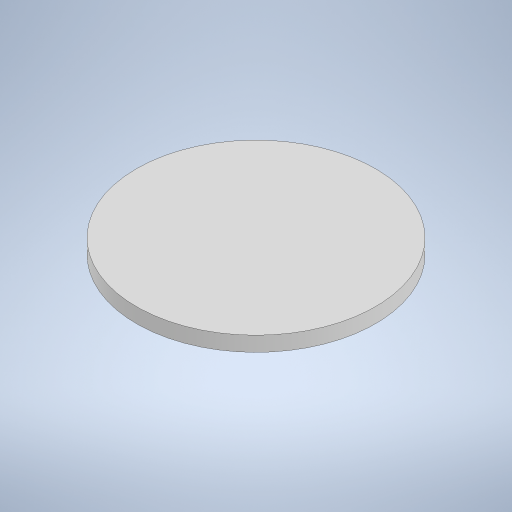
# Autodesk Inventor part: flow director r1
Saved by Autodesk Inventor 2024.1 (Build 281209000, 209)
## iProperties
Created: 2024-08-24
Part Number: flow director r1
Material: Generic
Document SubType Name: Modeling
Designer: pab2
Density: 1 g/cm^3
Appearance: Default
Author: pab2
Autodesk Inventor part; units mm, degrees
ref_plane "YZ Plane" through (0, 0, 0) normal (1, 0, 0) x (0, 1, 0)
ref_plane "XZ Plane" through (0, 0, 0) normal (0, 1, 0) x (-1, 0, 0)
ref_plane "XY Plane" through (0, 0, 0) normal (0, 0, 1) x (1, 0, 0)
sketch "Sketch1" plane through (0, 0, 0) normal (0, 1, 0) x (-1, 0, 0)
  circle A0 centre (0, 0) radius 12.7
  dimension "d0" = 25.4
  constraints: 1 centre point, 1 coincident
  measures "d0" diameter of A0
extrude "Extrusion1" add sketch "Sketch1" along normal blind 1.5748
sketch "Sketch2" plane through (0, 0, 0) normal (0, -1, 0) x (1, 0, 0)
  circle A0 centre (0, 0) radius 9.271
  line L0 (0, -9.271) -> (0, -7.271)
  line L1 (9.271, 0) -> (8.271, 0)
  line L2 (8.271, 0) -> (7.771, 0)
  line L3 (7.771, 0) -> (6.771, 0)
  line L4 (6.771, 0) -> (6.271, 0)
  line L5 (6.271, 0) -> (5.271, 0)
  line L6 (5.271, 0) -> (4.771, 0)
  line L7 (4.771, 0) -> (3.771, 0)
  line L8 (3.771, 0) -> (3.271, 0)
  line L9 (3.271, 0) -> (2.271, 0)
  line L10 (2.271, 0) -> (1.771, 0)
  line L11 (1.771, 0) -> (0.771, 0)
  line L12 (0.771, 0) -> (0.271, 0)
  line L13 (0, 9.271) -> (0, 7.271)
  circle A1 centre (0, 9.271) radius 1
  circle A2 centre (0, -9.271) radius 1
  circle A3 centre (5.7519, 7.271) radius 1
  line L14 (0, 0) -> (-0.5, 0)
  line L15 (-0.5, 0) -> (-1, 0)
  line L16 (-1, 0) -> (-2, 0)
  line L17 (-2, 0) -> (-2.5, 0)
  line L18 (-2.5, 0) -> (-3.5, 0)
  line L19 (-3.5, 0) -> (-4, 0)
  line L20 (-4, 0) -> (-5, 0)
  line L21 (-5, 0) -> (-5.5, 0)
  line L22 (-5.5, 0) -> (-6.5, 0)
  line L23 (-6.5, 0) -> (-7, 0)
  line L24 (-7, 0) -> (-8, 0)
  arc A4 (0, -9.271) -> (5.7519, 7.271) centre (-1.7377, 0.6042) ccw
  arc A5 (0, -9.271) -> (5.7519, 7.271) centre (-2.8108, 0.9773) ccw
  arc A6 (0, -9.271) -> (5.7519, 7.271) centre (-5.6528, 1.9656) ccw
  arc A7 (0, -9.271) -> (5.7519, 7.271) centre (-7.6502, 2.6601) ccw
  arc A8 (0, -9.271) -> (5.7519, 7.271) centre (-14.2057, 4.9395) ccw
  arc A9 (0, -9.271) -> (5.7519, 7.271) centre (-20.4184, 7.0998) ccw
  arc A10 (0, -9.271) -> (5.7519, 7.271) centre (-65.5254, 22.784) ccw
  arc A11 (0, -9.271) -> (5.7519, 7.271) centre (-794.5968, 276.2917) ccw
  arc A12 (5.7519, 7.271) -> (0, -9.271) centre (42.405, -14.7448) ccw
  arc A13 (5.7519, 7.271) -> (0, -9.271) centre (28.5048, -9.9115) ccw
  arc A14 (5.7519, 7.271) -> (0, -9.271) centre (17.401, -6.0506) ccw
  arc A15 (5.7519, 7.271) -> (0, -9.271) centre (14.5425, -5.0566) ccw
  arc A16 (5.7519, 7.271) -> (0, -9.271) centre (11.5077, -4.0014) ccw
  arc A17 (5.7519, 7.271) -> (0, -9.271) centre (10.0566, -3.4968) ccw
  arc A18 (5.7519, 7.271) -> (0, -9.271) centre (7.8443, -2.7276) ccw
  arc A19 (5.7519, 7.271) -> (0, -9.271) centre (6.9625, -2.4209) ccw
  arc A20 (5.7519, 7.271) -> (0, -9.271) centre (5.4808, -1.9057) ccw
  arc A21 (5.7519, 7.271) -> (0, -9.271) centre (4.8418, -1.6836) ccw
  arc A22 (5.7519, 7.271) -> (0, -9.271) centre (3.7059, -1.2886) ccw
  arc A23 (5.7519, 7.271) -> (0, -9.271) centre (3.1926, -1.1101) ccw
  arc A24 (5.7519, 7.271) -> (0, -9.271) centre (2.2472, -0.7814) ccw
  arc A25 (5.7519, 7.271) -> (0, -9.271) centre (1.8072, -0.6284) ccw
  line L25 (-8, 0) -> (-8.5, 0)
  arc A26 (5.7519, 7.271) -> (0, -9.271) centre (0.9779, -0.34) ccw
  arc A27 (5.7519, 7.271) -> (0, -9.271) centre (0.5844, -0.2032) ccw
  point P0 (-0.8639, 8.7673)
  point P1 (-0.9929, -9.1519)
  point P2 (-0.9865, -9.107)
  point P3 (-0.6349, 8.4984)
  point P4 (0, 8.0143)
  point P5 (-0.9657, -9.0112)
  point P6 (-0.9506, -8.9605)
  point P7 (0, 7.7083)
  point P8 (4.7804, 7.508)
  point P9 (-0.909, -8.8541)
  point P10 (-0.8816, -8.7991)
  point P11 (4.7676, 7.4478)
  point P12 (4.7529, 7.3167)
  point P13 (-0.8118, -8.6871)
  point P14 (-0.7685, -8.6312)
  point P15 (4.7522, 7.246)
  point P16 (4.7672, 7.0964)
  point P17 (-0.6639, -8.5232)
  point P18 (-0.6022, -8.4727)
  point P19 (4.7843, 7.0185)
  point P20 (4.8402, 6.8601)
  point P21 (-0.4601, -8.3831)
  point P22 (-0.3801, -8.3461)
  point P23 (4.8799, 6.7814)
  point P24 (4.9573, 6.6638)
  point P25 (-0.2465, -8.3019)
  point P26 (-0.1541, -8.2829)
  point P27 (5.018, 6.5917)
  point P28 (5.1633, 6.4625)
  point P29 (0.04, -8.2718)
  point P30 (0.1396, -8.2808)
  point P31 (5.247, 6.4078)
  point P32 (5.4327, 6.3233)
  point P33 (0.3376, -8.3297)
  point P34 (0.4333, -8.3697)
  point P35 (5.5325, 6.2954)
  point P36 (5.7393, 6.2711)
  point P37 (0.6105, -8.479)
  point P38 (0.6894, -8.5466)
  point P39 (5.8432, 6.2752)
  point P40 (6.0436, 6.3145)
  point P41 (0.8222, -8.7019)
  point P42 (0.8748, -8.7864)
  point P43 (6.1373, 6.3483)
  point P44 (0.9509, -8.9614)
  point P45 (0.975, -9.0488)
  point P46 (6.3787, 6.4918)
  point P47 (6.3055, 6.4383)
  dimension "d19" = 2
  dimension "d3" = 18.542
  dimension "d4" = 2
  dimension "d5" = 1
  dimension "d6" = 0.5
  dimension "d7" = 1
  dimension "d8" = 0.5
  dimension "d9" = 1
  dimension "d10" = 0.5
  dimension "d11" = 1
  dimension "d12" = 0.5
  dimension "d13" = 1
  dimension "d14" = 0.5
  dimension "d15" = 1
  dimension "d16" = 0.5
  dimension "d17" = 2
  dimension "d18" = 2
  dimension "d22" = 2
  dimension "d23" = 0.5
  dimension "d24" = 0.5
  dimension "d25" = 1
  dimension "d26" = 180
  dimension "d27" = 0.5
  dimension "d28" = 1
  dimension "d29" = 0.5
  dimension "d30" = 1
  dimension "d31" = 0.5
  dimension "d32" = 1
  dimension "d33" = 0.5
  dimension "d34" = 1
  dimension "d35" = 0.5
  constraints: 52 end point, 20 point on line, 5 point on circle, 3 centre point, 3 coincident, 3 horizontal, 2 vertical, 1 collinear, 99 other
  measures "d3" diameter of A0
  measures "d4" distance of L0.start L0.end
  measures "d5" distance of L1.start L1.end
  measures "d6" distance of L1.end L2.end
  measures "d7" distance of L2.end L3.end
  measures "d8" distance of L3.end L4.end
  measures "d9" distance of L4.end L5.end
  measures "d10" distance of L5.end L6.end
  measures "d11" distance of L6.end L7.end
  measures "d12" distance of L7.end L8.end
  measures "d13" distance of L8.end L9.end
  measures "d14" distance of L9.end L10.end
  measures "d15" distance of L10.end L11.end
  measures "d16" distance of L11.end L12.end
  measures "d17" distance of L13.start L13.end
  measures "d18" diameter of A1
  measures "d22" diameter of A3
  measures "d23" distance of L14.start L14.end
  measures "d24" distance of L14.end L15.end
  measures "d25" distance of L15.end L16.end
  measures "d26" angle of L16 L15
  measures "d27" distance of L16.end L17.end
  measures "d28" distance of L17.end L18.end
  measures "d29" distance of L18.end L19.end
  measures "d30" distance of L19.end L20.end
  measures "d31" distance of L20.end L21.end
  measures "d32" distance of L21.end L22.end
  measures "d33" distance of L22.end L23.end
  measures "d34" distance of L23.end L24.end
  measures "d35" distance of L24.end L25.end
extrude "Extrusion2" add sketch "Sketch2" along normal blind 1.8 contours A4 A2 A5 L2 | L2 A5 A3 A4 | A6 L4 A7 A3 | A8 L6 A9 A3 | A10 L8 A11 A3 | A12 L10 A13 A3 | A14 L12 A15 A3 | A16 L15 A17 A3 | A18 L17 A19 A3 | A20 L19 A21 A3 | A22 L21 A23 A3 | A2 A7 L4 A6 | A2 A9 L6 A8 | A2 A11 L8 A10 | A2 A13 L10 A12 | A2 A15 L12 A14 | A2 A17 L15 A16 | A2 A19 L17 A18 | A2 A21 L19 A20 | A2 A23 L21 A22 | A2 A25 L23 A24 | A2 A27 L25 A26 | A24 L23 A25 L13 | L25 A27 A1 A26
sketch "Sketch3" plane through (0, 0, 0) normal (0, -1, 0) x (1, 0, 0)
  point P0 (0, 0)
body "Solid1"
